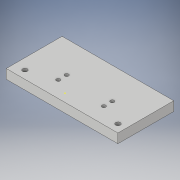
# Autodesk Inventor part: servostand
Saved by Autodesk Inventor 2019 (Build 230136000, 136)
## iProperties
Created: 2020-02-26
Part Number: servostand
Material: Generic
Document SubType Name: Modeling
Designer: Hp
Density: 1 g/cm^3
Appearance: Default
Author: Hp
Autodesk Inventor part; units mm, degrees
ref_plane "YZ Plane" through (0, 0, 0) normal (1, 0, 0) x (0, 1, 0)
ref_plane "XZ Plane" through (0, 0, 0) normal (0, 1, 0) x (-1, 0, 0)
ref_plane "XY Plane" through (0, 0, 0) normal (0, 0, 1) x (1, 0, 0)
sketch "Sketch1" plane through (0, 0, 0) normal (0, 1, 0) x (-1, 0, 0)
  line L0 (54.4765, 8.5395) -> (-65.5235, 8.5395)
  line L1 (-65.5235, 8.5395) -> (-65.5235, -51.4605)
  line L2 (-65.5235, -51.4605) -> (54.4765, -51.4605)
  line L3 (54.4765, -51.4605) -> (54.4765, 8.5395)
  line L4 (42.9455, 0) -> (-57.0545, 0)
  circle A0 centre (42.9455, 0) radius 2.5
  circle A1 centre (-57.0545, 0) radius 2.5
  point P0 (0, 0)
  dimension "d0" = 120
  dimension "d1" = 60
  dimension "d2" = 100
  dimension "d3" = 5
  dimension "d4" = 5
  constraints: 10 end point, 2 centre point, 2 coincident, 2 horizontal, 2 parallel, 1 perpendicular
  measures "d0" distance of L2.end L1.end
  measures "d1" distance of L1.end L0.end
  measures "d2" distance of L4.start L4.end
  measures "d3" diameter of A0
  measures "d4" diameter of A1
extrude "Extrusion1" add sketch "Sketch1" along normal blind 10
sketch "Sketch2" plane through (0, 10, 0) normal (0, 1, 0) x (1, 0, 0)
  line L0 (-16.1382, 5.2435) -> (17.0718, 5.2435)
  circle A0 centre (-16.1382, 5.2435) radius 1
  circle A1 centre (17.0718, 5.2435) radius 1
  point P0 (0, 0)
  dimension "d7" = 33.21
  dimension "d8" = 2
  dimension "d9" = 2
  constraints: 2 centre point, 2 coincident, 2 end point, 1 horizontal
  measures "d7" distance of L0.start L0.end
  measures "d8" diameter of A0
  measures "d9" diameter of A1
extrude "Extrusion2" cut sketch "Sketch2" along normal blind 10
sketch "Sketch3" plane through (0, 10, 0) normal (0, 1, 0) x (1, 0, 0)
  point P0 (0, 0)
sketch "Sketch4" plane through (0, 10, 0) normal (0, 1, 0) x (1, 0, 0)
  circle A0 centre (-16.1382, 5.2435) radius 1 projected
  circle A1 centre (30.8669, 5.2794) radius 1
  point P0 (0, 0)
  dimension "d13" = 2
  constraints: 1 centre point
  measures "d13" diameter of A1
extrude "Extrusion3" cut sketch "Sketch4" along normal blind 10 contours A1
sketch "Sketch5" plane through (0, 10, 0) normal (0, 1, 0) x (1, 0, 0)
  circle A0 centre (-16.1382, 5.2435) radius 1 projected
  circle A1 centre (30.8669, 5.2794) radius 1 projected
  circle A2 centre (30.8669, 14.2341) radius 2
  circle A3 centre (-16.1382, 14.2341) radius 2
  point P0 (0, 0)
  dimension "d20" = 4
  dimension "d21" = 4
  constraints: 2 centre point
  measures "d20" diameter of A2
  measures "d21" diameter of A3
extrude "Extrusion4" cut sketch "Sketch5" along normal blind 10 contours A2 | A3
sketch "Sketch6" plane through (0, 10, 0) normal (0, 1, 0) x (1, 0, 0)
  circle A0 centre (-15.9518, 8.8125) radius 2
  circle A1 centre (33.0446, 8.8125) radius 2
  circle A2 centre (-15.9518, 17.8231) radius 2
  circle A3 centre (33.0446, 17.8231) radius 2
  point P0 (0, 0)
  dimension "d24" = 4
  dimension "d26" = 4
  dimension "d30" = 4
  constraints: 4 centre point
  measures "d24" diameter of A0
  measures "d26" diameter of A1
  measures "d30" diameter of A2
extrude "Extrusion5" cut sketch "Sketch6" against normal blind 10
body "Solid1"
